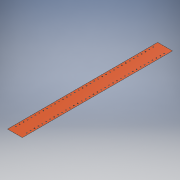
# Autodesk Inventor part: Skin NPS 18 Internal
Saved by Autodesk Inventor 2019 (Build 230136000, 136)
## iProperties
Created: 2016-08-30
Part Number: Skin NPS 18 Internal
Material: Rubber, Silicone
Document SubType Name: Modeling
Designer: IEUser
Density: 1.25 g/cm^3
Appearance: Rubber - Black
Author: IEUser
Autodesk Inventor part; units mm, degrees
ref_plane "YZ Plane" through (0, 0, 0) normal (1, 0, 0) x (0, 1, 0)
ref_plane "XZ Plane" through (0, 0, 0) normal (0, 1, 0) x (-1, 0, 0)
ref_plane "XY Plane" through (0, 0, 0) normal (0, 0, 1) x (1, 0, 0)
sketch "Skin Scheme" plane through (0, 0, 0) normal (0, 1, 0) x (-1, 0, 0)
  line L0 (909.5, -84.5) -> (-909.5, -84.5)
  line L1 (-909.5, -84.5) -> (-909.5, 84.5)
  line L2 (-909.5, 84.5) -> (909.5, 84.5)
  line L3 (909.5, 84.5) -> (909.5, -84.5)
  circle A0 centre (787.5, -62.5) radius 5
  circle A1 centre (742.5, -62.5) radius 5
  circle A2 centre (697.5, -62.5) radius 5
  circle A3 centre (652.5, -62.5) radius 5
  circle A4 centre (607.5, -62.5) radius 5
  circle A5 centre (562.5, -62.5) radius 5
  circle A6 centre (517.5, -62.5) radius 5
  circle A7 centre (472.5, -62.5) radius 5
  circle A8 centre (427.5, -62.5) radius 5
  circle A9 centre (382.5, -62.5) radius 5
  circle A10 centre (337.5, -62.5) radius 5
  circle A11 centre (292.5, -62.5) radius 5
  circle A12 centre (247.5, -62.5) radius 5
  circle A13 centre (202.5, -62.5) radius 5
  circle A14 centre (157.5, -62.5) radius 5
  circle A15 centre (112.5, -62.5) radius 5
  circle A16 centre (67.5, -62.5) radius 5
  circle A17 centre (22.5, -62.5) radius 5
  circle A18 centre (787.5, 62.5) radius 5
  circle A19 centre (742.5, 62.5) radius 5
  circle A20 centre (697.5, 62.5) radius 5
  circle A21 centre (652.5, 62.5) radius 5
  circle A22 centre (607.5, 62.5) radius 5
  circle A23 centre (562.5, 62.5) radius 5
  circle A24 centre (517.5, 62.5) radius 5
  circle A25 centre (472.5, 62.5) radius 5
  circle A26 centre (427.5, 62.5) radius 5
  circle A27 centre (382.5, 62.5) radius 5
  circle A28 centre (337.5, 62.5) radius 5
  circle A29 centre (292.5, 62.5) radius 5
  circle A30 centre (247.5, 62.5) radius 5
  circle A31 centre (202.5, 62.5) radius 5
  circle A32 centre (157.5, 62.5) radius 5
  circle A33 centre (112.5, 62.5) radius 5
  circle A34 centre (67.5, 62.5) radius 5
  circle A35 centre (22.5, 62.5) radius 5
  circle A36 centre (-22.5, -62.5) radius 5
  circle A37 centre (-22.5, 62.5) radius 5
  circle A38 centre (-67.5, -62.5) radius 5
  circle A39 centre (-67.5, 62.5) radius 5
  circle A40 centre (-112.5, -62.5) radius 5
  circle A41 centre (-112.5, 62.5) radius 5
  circle A42 centre (-157.5, -62.5) radius 5
  circle A43 centre (-157.5, 62.5) radius 5
  circle A44 centre (-202.5, -62.5) radius 5
  circle A45 centre (-202.5, 62.5) radius 5
  circle A46 centre (-247.5, -62.5) radius 5
  circle A47 centre (-247.5, 62.5) radius 5
  circle A48 centre (-292.5, -62.5) radius 5
  circle A49 centre (-292.5, 62.5) radius 5
  circle A50 centre (-337.5, -62.5) radius 5
  circle A51 centre (-337.5, 62.5) radius 5
  circle A52 centre (-382.5, -62.5) radius 5
  circle A53 centre (-382.5, 62.5) radius 5
  circle A54 centre (-427.5, -62.5) radius 5
  circle A55 centre (-427.5, 62.5) radius 5
  circle A56 centre (-472.5, -62.5) radius 5
  circle A57 centre (-472.5, 62.5) radius 5
  circle A58 centre (-517.5, -62.5) radius 5
  circle A59 centre (-517.5, 62.5) radius 5
  circle A60 centre (-562.5, -62.5) radius 5
  circle A61 centre (-562.5, 62.5) radius 5
  circle A62 centre (-607.5, -62.5) radius 5
  circle A63 centre (-607.5, 62.5) radius 5
  circle A64 centre (-652.5, -62.5) radius 5
  circle A65 centre (-652.5, 62.5) radius 5
  circle A66 centre (-697.5, -62.5) radius 5
  circle A67 centre (-697.5, 62.5) radius 5
  circle A68 centre (-742.5, -62.5) radius 5
  circle A69 centre (-742.5, 62.5) radius 5
  circle A70 centre (-787.5, -62.5) radius 5
  circle A71 centre (-787.5, 62.5) radius 5
  point P0 (0, 0)
  dimension "d0" = 1819
  dimension "d1" = 909.5
  dimension "d2" = 169
  dimension "d3" = 84.5
  dimension "d4" = 10
  dimension "d5" = 122
  dimension "d6" = 22
  dimension "d9" = 45
  dimension "d12" = 125
  constraints: 72 centre point, 8 end point, 2 horizontal, 2 parallel, 1 perpendicular, 1 vertical, 142 other
  measures "d0" distance of L0.start L0.end
  measures "d1" distance from line of point (0, 0) L3
  measures "d2" distance of L2.end L0.start
  measures "d3" distance from line of point (0, 0) L0
  measures "d4" diameter of A0
  measures "d5" distance from line of L3 A0.centre
  measures "d6" distance from line of L0 A0.centre
  measures "d9" distance of A0.centre A1.centre
  measures "d12" distance of A0.centre A18.centre
extrude "Skin Body" add sketch "Skin Scheme" along normal blind 1
sketch "End Cut Outline" plane through (0, 1, 0) normal (0, 1, 0) x (1, 0, 0)
  line L0 (-859.5, 94.5) -> (-919.5, 94.5)
  line L1 (-919.5, 94.5) -> (-919.5, -94.5)
  line L2 (-919.5, -94.5) -> (-859.5, -94.5)
  line L3 (-859.5, -94.5) -> (-859.5, 94.5)
  line L4 (909.5, 84.5) -> (-909.5, 84.5) projected
  line L5 (-909.5, -84.5) -> (909.5, -84.5) projected
  line L6 (-909.5, 84.5) -> (-909.5, -84.5) projected
  point P0 (0, 0)
  dimension "d19" = 10
  dimension "d20" = 10
  dimension "d21" = 10
  dimension "d22" = 50
  constraints: 8 end point, 2 parallel, 1 horizontal, 1 perpendicular
  measures "d19" distance between parallel lines of L4 L0
  measures "d20" distance between parallel lines of L5 L2
  measures "d21" distance between parallel lines of L6 L1
  measures "d22" distance between parallel lines of L3 L6
extrude "End Cut" cut sketch "End Cut Outline" along normal through all both and the other way through all
mirror "End Cut Mirror" about plane through (0, 0, 0) normal (1, 0, 0) of "End Cut"
equation "\"d1\" = 0.5 * d0"
equation "\"d3\" = 0.5 * d2"
body "Solid2"
